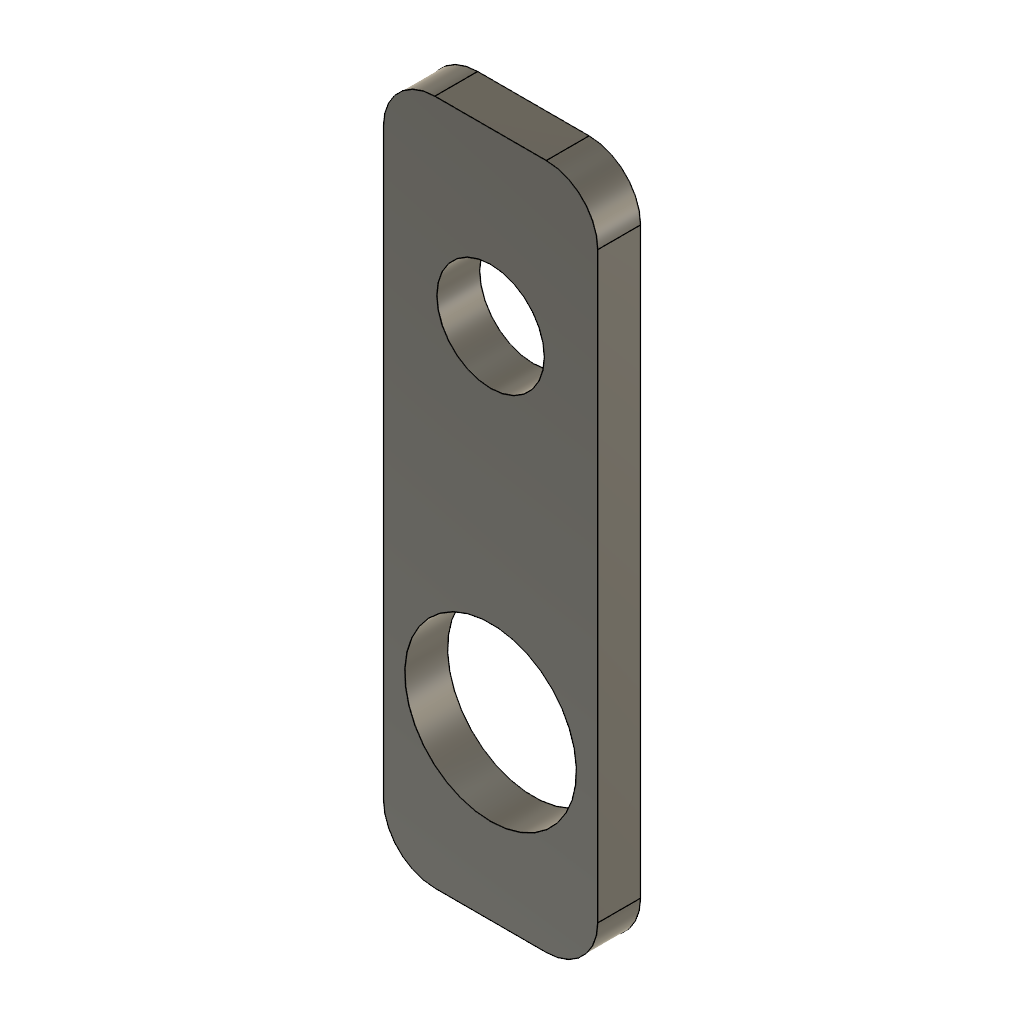
BracketLink (Autodesk Fusion 360 design; units mm, degrees)
part number: 2026-10-01-01-08-11-639
Autodesk Fusion 360 part; units mm, degrees
sketch "Sketch1" plane through (0, 0, 0) normal (0, 1, 0) x (1, 0, 0)
  line L0 (-6.35, -50.8) -> (25.4, -50.8)
  line L1 (25.4, -50.8) -> (25.4, 50.8)
  line L2 (25.4, 50.8) -> (-6.35, 50.8)
  line L3 (-6.35, 50.8) -> (-6.35, -50.8)
  dimension "d6" = 31.75
  dimension "d7" = 101.6
  constraint horizontal L0
  constraint vertical L1
  constraint horizontal L2
  constraint vertical L3
  measures "d6" distance of L1.end L2.end
  measures "d7" distance of L0.start L2.end
extrude "Extrude1" add sketch "Sketch1" along normal blind 6.35
hole "Hole1" at (9.525, 0, 25.4) direction (0, 1, 0) diameter 15.9004 depth 12.7 tip angle 118
hole "Hole2" at (9.525, 0, -25.4) direction (0, 1, 0) diameter 25.4 depth 12.7 tip angle 118
fillet "Fillet1" radius 7.62 1 edges at (25.4, 3.175, 50.8)
fillet "Fillet2" radius 7.62 1 edges at (-6.35, 3.175, 50.8)
fillet "Fillet3" radius 7.62 1 edges at (25.4, 3.175, -50.8)
fillet "Fillet4" radius 7.62 1 edges at (-6.35, 3.175, -50.8)
equation "Fit_Height = 4.00 in"
equation "Fit_Length = 1.25 in"
equation "Fit_Width = 0.25 in"
equation "Hole_D1 = 0.626 in"
equation "Hole_D2 = 1.00 in"
equation "d6 = Fit_Length"
equation "d7 = Fit_Height"
equation "d8 = Fit_Width"
equation "d11 = Hole_D1"
equation "d16 = Hole_D2"
